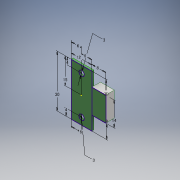
# Autodesk Inventor part: sensor
Saved by Autodesk Inventor 2018.3 (Build 223284000, 284)
## iProperties
Created: 2019-09-27
Part Number: sensor
Material: 一般
Document SubType Name: Modeling
Designer: Eiji Nishizawa
Density: 1 g/cm^3
Appearance: 滑らか - 濃い深緑
Author: Eiji Nishizawa
Autodesk Inventor part; units mm, degrees
ref_plane "YZ Plane" through (0, 0, 0) normal (1, 0, 0) x (0, 1, 0)
ref_plane "XZ Plane" through (0, 0, 0) normal (0, 1, 0) x (-1, 0, 0)
ref_plane "XY Plane" through (0, 0, 0) normal (0, 0, 1) x (1, 0, 0)
sketch "スケッチ1" plane through (0, 0, 0) normal (0, 1, 0) x (-1, 0, 0)
  line L0 (6, 15) -> (-6, 15)
  line L1 (-6, 15) -> (-6, -15)
  line L2 (-6, -15) -> (6, -15)
  line L3 (6, -15) -> (6, 15)
  line L4 (-6, 7) -> (-14, 7)
  line L5 (-14, 7) -> (-14, -7)
  line L6 (-14, -7) -> (-6, -7)
  line L7 (-6, -7) -> (-6, 7)
  circle A0 centre (0, 11) radius 1.5
  circle A1 centre (0, -11) radius 1.5
  point P0 (0, 0)
  dimension "d0" = 30
  dimension "d1" = 12
  dimension "d2" = 14
  dimension "d3" = 8
  dimension "d4" = 8
  dimension "d5" = 15
  dimension "d6" = 6
  dimension "d7" = 8
  dimension "d8" = 3
  dimension "d9" = 3
  dimension "d10" = 6
  dimension "d11" = 6
  dimension "d12" = 4
  dimension "d13" = 4
  constraints: 16 end point, 4 parallel, 2 centre point, 2 horizontal, 2 perpendicular, 1 point on line
  measures "d0" distance between parallel lines of L2 L0
  measures "d1" distance of L0.start L0.end
  measures "d2" distance between parallel lines of L6 L4
  measures "d3" distance between parallel lines of L2 L6
  measures "d4" distance between parallel lines of L0 L4
  measures "d5" distance from line of point (0, 0) L0
  measures "d6" distance from line of L1 point (0, 0)
  measures "d7" distance between parallel lines of L5 L1
  measures "d8" diameter of A0
  measures "d9" diameter of A1
  measures "d10" distance from line of L3 A0.centre
  measures "d11" distance from line of L3 A1.centre
  measures "d12" distance from line of L2 A1.centre
  measures "d13" distance from line of L0 A0.centre
extrude "押し出し1" add sketch "スケッチ1" along normal blind 1.2 contours L3 L2 L1 L0
extrude "押し出し2" add sketch "スケッチ1" along normal blind 5 contours L1 L6 L5 L4
sketch "スケッチ2" plane through (0, 1.2, 0) normal (0, 1, 0) x (1, 0, 0)
  line L0 (-1, -2) -> (1, -2)
  line L1 (1, -2) -> (1, 2)
  line L2 (1, 2) -> (-1, 2)
  line L3 (-1, 2) -> (-1, -2)
  point P0 (0, 0)
  dimension "d18" = 2
  dimension "d19" = 4
  dimension "d20" = 2
  dimension "d21" = 1
  constraints: 8 end point, 2 parallel, 1 horizontal, 1 perpendicular
  measures "d18" distance between parallel lines of L1 L3
  measures "d19" distance between parallel lines of L2 L0
  measures "d20" distance from line of point (0, 0) L2
  measures "d21" distance from line of L1 point (0, 0)
extrude "押し出し3" add sketch "スケッチ2" along normal blind 1.2
